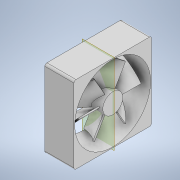
# Autodesk Inventor part: radiator_fan
Saved by Autodesk Inventor 2020 (Build 240168000, 168)
## iProperties
Created: 2022-08-31
Part Number: radiator_fan
Material: Generic
Document SubType Name: Modeling
Designer: Intuito_PC
Density: 1 g/cm^3
Appearance: Default
Author: Intuito_PC
Autodesk Inventor part; units mm, degrees
ref_plane "YZ Plane" through (0, 0, 0) normal (1, 0, 0) x (0, 1, 0)
ref_plane "XZ Plane" through (0, 0, 0) normal (0, 1, 0) x (-1, 0, 0)
ref_plane "XY Plane" through (0, 0, 0) normal (0, 0, 1) x (1, 0, 0)
sketch "Sketch1" plane through (0, 0, 0) normal (1, 0, 0) x (0, 1, 0)
  line L0 (0, 0) -> (120, 0)
  line L1 (120, 0) -> (120, 120)
  line L2 (120, 120) -> (0, 120)
  line L3 (0, 120) -> (0, 0)
  dimension "d0" = 120
  dimension "d1" = 120
  constraints: 8 end point, 2 parallel, 1 horizontal, 1 perpendicular
  measures "d0" distance of L2.end L1.end
  measures "d1" distance of L1.end L0.end
extrude "Extrusion1" add sketch "Sketch1" along normal blind 45
fillet "Fillet1" radius 3.175 4 edges at (22.5, 120, 120) (22.5, 120, 0) (22.5, 0, 120) (22.5, 0, 0)
sketch "Sketch2" plane through (45, 0, 0) normal (1, 0, 0) x (0, 0, -1)
  line L0 (-60, 60) -> (-60, 59.8888)
  circle A0 centre (-60, 59.8888) radius 58.6654
  point P0 (0, 0)
  constraints: 2 end point, 1 centre point, 1 coincident, 1 vertical
extrude "Extrusion2" cut sketch "Sketch2" against normal blind 45
ref_plane "Work Plane1" through (0, 3.175, 60) normal (0, 0, -1) x (-1, 0, 0)
sketch "Sketch3" plane through (0, 3.175, 60) normal (0, 0, -1) x (-1, 0, 0)
  arc A0 (-1.7704, 85.4358) -> (-40.8454, 56.825) centre (27.4593, 4.527) ccw
  arc A1 (-1.0909, 83.5548) -> (-39.2574, 55.6091) centre (27.4593, 4.527) ccw
  line L0 (-40.8454, 56.825) -> (-39.0774, 55.8433)
  line L1 (-1.0909, 83.5548) -> (-1.7704, 85.4358)
  point P0 (0, -3.175)
  dimension "d8" = 2
  constraints: 5 point on circle, 4 end point, 2 centre point
  measures "d8" radial gap between concentric circles of A0 A1
extrude "Extrusion3" add sketch "Sketch3" along normal blind 48.26
sketch "Sketch4" plane through (0, 3.175, 60) normal (0, 0, -1) x (-1, 0, 0)
  arc A0 (-1.7704, 85.4358) -> (-40.8454, 56.825) centre (27.4593, 4.527) ccw projected
  line L0 (-40.8454, 56.825) -> (-4.8465, 56.825)
  point P0 (0, -3.175)
  constraints: 2 end point, 1 horizontal
pattern_circular "Circular Pattern1" count 6 over 360 about axis through (45, 59.8888, 60) along (-1, 0, 0) of "Extrusion3"
sketch "Sketch5" plane through (45, 0, 0) normal (1, 0, 0) x (0, 0, -1)
  circle A0 centre (-59.8691, 59.7266) radius 15.4187
  point P0 (0, 0)
  constraints: 1 centre point
extrude "Extrusion4" add sketch "Sketch5" against normal blind 45
body "Solid1"
